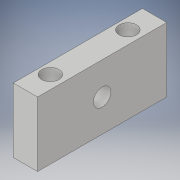
# Autodesk Inventor part: WheelIntakeSpringStop
Saved by Autodesk Inventor 2017 (Build 210142000, 142)
## iProperties
Created: 2018-01-03
Part Number: WheelIntakeSpringStop
Material: Generic
Document SubType Name: Modeling
Designer: User
Density: 1 g/cm^3
Appearance: Default
Author: User
Autodesk Inventor part; units mm, degrees
ref_plane "YZ Plane" through (0, 0, 0) normal (1, 0, 0) x (0, 1, 0)
ref_plane "XZ Plane" through (0, 0, 0) normal (0, 1, 0) x (-1, 0, 0)
ref_plane "XY Plane" through (0, 0, 0) normal (0, 0, 1) x (1, 0, 0)
sketch "Sketch1" plane through (0, 0, 0) normal (1, 0, 0) x (0, 1, 0)
  line L0 (0, 0) -> (12.7, 0)
  line L1 (12.7, 0) -> (12.7, -25.4)
  line L2 (12.7, -25.4) -> (0, -25.4)
  line L3 (0, -25.4) -> (0, 0)
  dimension "d0" = 12.7
  dimension "d1" = 25.4
  constraints: 8 end point, 2 parallel, 1 horizontal, 1 perpendicular
  measures "d0" distance of L1.end L2.end
  measures "d1" distance of L0.end L1.end
extrude "Extrusion1" add sketch "Sketch1" along normal blind 4.7752
sketch "Sketch2" plane through (0, 12.7, 0) normal (0, 1, 0) x (1, 0, 0)
  line L0 (0, 25.4) -> (4.7752, 25.4) projected
  line L1 (0, 0) -> (4.7752, 0) projected
  point P0 (2.2104, 5.08)
  point P1 (2.2104, 20.32)
  dimension "d22" = 5.08
  dimension "d23" = 5.08
  measures "d22" distance from line of point (2.21, 20.32) L0
  measures "d23" distance from line of L1 point (2.21, 5.08)
hole "Hole1" at (2.2104, 12.7, -5.08) at (2.2104, 12.7, -20.32) direction (0, -1, 0) diameter 3.429 end through all
sketch "Sketch3" plane through (0, 0, 0) normal (-1, 0, 0) x (0, 0, 1)
  line L0 (0, 12.7) -> (-25.4, 12.7) projected
  line L1 (-25.4, 0) -> (0, 0) projected
  line L2 (0, 0) -> (0, 12.7) projected
  point P0 (-12.7, 6.35)
  dimension "d11" = 12.7
  dimension "d12" = 25.4
  dimension "d13" = 6.35
  dimension "d14" = 12.7
  measures "d11" distance between parallel lines of L0 L1
  measures "d12" distance of L1.start L1.end
  measures "d13" distance from line of L1 point (-12.7, 6.35)
  measures "d14" distance from line of L2 point (-12.7, 6.35)
hole "Hole2" at (0, 6.35, -12.7) direction (1, 0, 0) diameter 3.429 end through all
equation "\"d13\" = 0.5 * d11"
body "Solid1"
